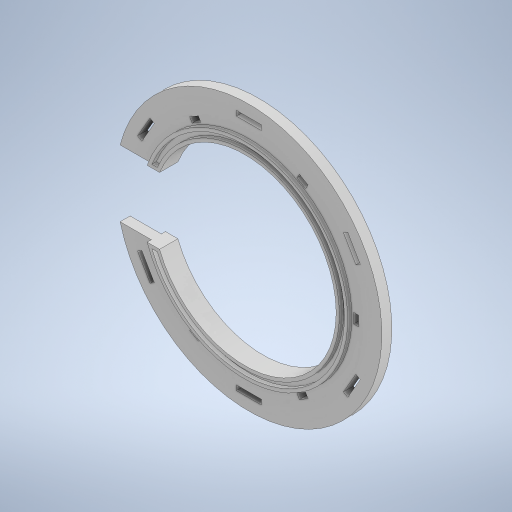
# Autodesk Inventor part: [3DP]back_cir_hold_final
Saved by Autodesk Inventor 2024 (Build 280153000, 153)
## iProperties
Created: 2024-03-23
Part Number: [3DP]back_cir_hold_final
Material: Generic
Document SubType Name: Modeling
Designer: op04o
Density: 1 g/cm^3
Appearance: Default
Author: op04o
Autodesk Inventor part; units mm, degrees
ref_plane "YZ Plane" through (0, 0, 0) normal (1, 0, 0) x (0, 1, 0)
ref_plane "XZ Plane" through (0, 0, 0) normal (0, 1, 0) x (-1, 0, 0)
ref_plane "XY Plane" through (0, 0, 0) normal (0, 0, 1) x (1, 0, 0)
sketch "Sketch1" plane through (0, 0, 0) normal (0, 0, 1) x (1, 0, 0)
  circle A0 centre (0, 0) radius 80
  circle A1 centre (0, 0) radius 55
  line L0 (-7.5, 73) -> (7.5, 73)
  line L1 (7.5, 73) -> (7.5, 70)
  line L2 (7.5, 70) -> (-7.5, 70)
  line L3 (-7.5, 70) -> (-7.5, 73)
  line L4 (-66.9699, 30.0048) -> (-59.4699, 42.9952)
  line L5 (-59.4699, 42.9952) -> (-56.8718, 41.4952)
  line L6 (-56.8718, 41.4952) -> (-64.3718, 28.5048)
  line L7 (-64.3718, 28.5048) -> (-66.9699, 30.0048)
  line L8 (-59.4699, -42.9952) -> (-66.9699, -30.0048)
  line L9 (-66.9699, -30.0048) -> (-64.3718, -28.5048)
  line L10 (-64.3718, -28.5048) -> (-56.8718, -41.4952)
  line L11 (-56.8718, -41.4952) -> (-59.4699, -42.9952)
  line L12 (7.5, -73) -> (-7.5, -73)
  line L13 (-7.5, -73) -> (-7.5, -70)
  line L14 (-7.5, -70) -> (7.5, -70)
  line L15 (7.5, -70) -> (7.5, -73)
  line L16 (66.9699, -30.0048) -> (59.4699, -42.9952)
  line L17 (59.4699, -42.9952) -> (56.8718, -41.4952)
  line L18 (56.8718, -41.4952) -> (64.3718, -28.5048)
  line L19 (64.3718, -28.5048) -> (66.9699, -30.0048)
  line L20 (59.4699, 42.9952) -> (66.9699, 30.0048)
  line L21 (66.9699, 30.0048) -> (64.3718, 28.5048)
  line L22 (64.3718, 28.5048) -> (56.8718, 41.4952)
  line L23 (56.8718, 41.4952) -> (59.4699, 42.9952)
  line L24 (-58.1708, 43.7452) -> (-43.1708, 43.7452)
  line L25 (-43.1708, 43.7452) -> (-43.1708, 40.7452)
  line L26 (-43.1708, 40.7452) -> (-58.1708, 40.7452)
  line L27 (-58.1708, 40.7452) -> (-58.1708, 43.7452)
  line L28 (-58.1708, -40.7452) -> (-43.1708, -40.7452)
  line L29 (-43.1708, -40.7452) -> (-43.1708, -43.7452)
  line L30 (-43.1708, -43.7452) -> (-58.1708, -43.7452)
  line L31 (-58.1708, -43.7452) -> (-58.1708, -40.7452)
  line L32 (0, 20) -> (-100, 20)
  line L33 (-100, 20) -> (-100, -20)
  line L34 (-100, -20) -> (0, -20)
  line L35 (0, -20) -> (0, 20)
  point P0 (0, 73)
  point P1 (7.5, 71.5)
  point P2 (0, 70)
  point P3 (-63.2199, 36.5)
  point P4 (-58.1708, 42.2452)
  point P5 (-60.6218, 35)
  point P6 (-63.2199, -36.5)
  point P7 (-65.6708, -29.2548)
  point P8 (-60.6218, -35)
  point P9 (0, -73)
  point P10 (-7.5, -71.5)
  point P11 (0, -70)
  point P12 (63.2199, -36.5)
  point P13 (58.1708, -42.2452)
  point P14 (60.6218, -35)
  point P15 (63.2199, 36.5)
  point P16 (65.6708, 29.2548)
  point P17 (60.6218, 35)
  point P18 (-58.1708, 42.2452)
  point P19 (-58.1708, -42.2452)
  point P20 (-51.2348, -20)
  point P21 (-77.4597, -20)
  point P22 (-77.4597, 20)
  point P23 (-51.2348, 20)
  dimension "d0" = 160
  dimension "d1" = 110
  dimension "d2" = 15
  dimension "d3" = 3
  dimension "d11" = 70
  dimension "d14" = 360
  dimension "d18" = 15
  dimension "d19" = 3
  dimension "d20" = 15
  dimension "d21" = 3
  dimension "d22" = 40
  dimension "d23" = 100
  constraints: 72 end point, 8 midpoint, 8 parallel, 4 horizontal, 4 perpendicular, 3 coincident, 2 centre point, 1 vertical alignment, 67 other
  measures "d0" diameter of A0
  measures "d1" diameter of A1
  measures "d2" distance of L1.end L2.end
  measures "d3" distance of L0.end L1.end
  measures "d11" distance of point (0, 0) point (0, 70)
  measures "d18" distance of L24.start L24.end
  measures "d19" distance of L24.end L25.end
  measures "d20" distance of L28.start L28.end
  measures "d21" distance of L30.end L28.start
  measures "d22" distance of L32.end L33.end
  measures "d23" distance of L32.start L32.end
extrude "Extrusion2" add sketch "Sketch1" along normal blind 6 contours A0 L34 A1 L32 | L27 L24 L25 L26 L6 L5 | L11 L10 L28 L29 L30 L31 picked at (16.7927, -65.9701)
sketch "草圖2" plane through (0, 0, 6) normal (0, 0, 1) x (1, 0, 0)
  arc A0 (-51.2348, -20) -> (-51.2348, 20) centre (0, 0) ccw projected
  circle A1 centre (0, 0) radius 55
  circle A2 centre (0, 0) radius 57
  circle A3 centre (0, 0) radius 60
  circle A4 centre (0, 0) radius 62
  arc A5 (-77.4597, -20) -> (-77.4597, 20) centre (0, 0) ccw projected
  line L0 (-51.2348, 20) -> (-77.4597, 20)
  line L1 (-51.2348, -20) -> (-77.4597, -20) projected
  line L2 (-51.2348, -20) -> (-77.4597, -20)
  line L3 (-51.2348, 20) -> (-77.4597, 20)
  line L4 (-77.4597, 20) -> (-77.4597, 22)
  line L5 (-77.4597, 22) -> (-51.2348, 22)
  line L6 (-51.2348, 22) -> (-51.2348, 20)
  line L7 (-77.4597, -20) -> (-51.2348, -20)
  line L8 (-51.2348, -20) -> (-51.2348, -22)
  line L9 (-51.2348, -22) -> (-77.4597, -22)
  line L10 (-77.4597, -22) -> (-77.4597, -20)
  point P0 (-58.6856, 20)
  point P1 (-58.6856, -20)
  point P2 (-55.8211, 22)
  point P3 (-55.8211, -22)
  point P4 (-52.5833, -22)
  point P5 (-52.5833, 22)
  dimension "d24" = 114
  dimension "d25" = 120
  dimension "d26" = 124
  dimension "d27" = 2
  dimension "d28" = 26.2249
  dimension "d29" = 2
  dimension "d30" = 26.2249
  constraints: 20 end point, 4 coincident, 4 horizontal, 4 parallel, 3 centre point, 2 perpendicular, 3 other
  measures "d24" diameter of A2
  measures "d25" diameter of A3
  measures "d26" diameter of A4
  measures "d27" distance of L3.end L4.end
  measures "d28" distance of L4.end L5.end
  measures "d29" distance of L7.end L8.end
  measures "d30" distance of L8.end L9.end
extrude "擠出3" add sketch "草圖2" against normal blind 8.5 contours L8 L9 A2 L1 | A0 L6 L5 A2 L9 L8 | L0 A2 L5 L6 | A2 L9 A3 L1 | L0 A3 L5 A2 | A3 L9 A4 L1 | L0 A4 L5 A3 | A3 L5 A4 L9
extrude "擠出4" add sketch "草圖2" along normal blind 2.5 contours L8 L9 A2 L1 | A0 L6 L5 A2 L9 L8 | L0 A2 L5 L6 | A2 L9 A3 L1 | L0 A3 L5 A2 | A3 L9 A4 L1 | L0 A4 L5 A3 | A3 L5 A4 L9
sketch "草圖3" plane through (0, 0, 6) normal (0, 0, 1) x (1, 0, 0)
  line L0 (63, 3) -> (66, 3)
  line L1 (66, 3) -> (66, -3)
  line L2 (66, -3) -> (63, -3)
  line L3 (63, -3) -> (63, 3)
  line L4 (28.9019, 56.0596) -> (30.4019, 58.6577)
  line L5 (30.4019, 58.6577) -> (35.5981, 55.6577)
  line L6 (35.5981, 55.6577) -> (34.0981, 53.0596)
  line L7 (34.0981, 53.0596) -> (28.9019, 56.0596)
  line L8 (-34.0981, 53.0596) -> (-35.5981, 55.6577)
  line L9 (-35.5981, 55.6577) -> (-30.4019, 58.6577)
  line L10 (-30.4019, 58.6577) -> (-28.9019, 56.0596)
  line L11 (-28.9019, 56.0596) -> (-34.0981, 53.0596)
  line L12 (-63, -3) -> (-66, -3)
  line L13 (-66, -3) -> (-66, 3)
  line L14 (-66, 3) -> (-63, 3)
  line L15 (-63, 3) -> (-63, -3)
  line L16 (-28.9019, -56.0596) -> (-30.4019, -58.6577)
  line L17 (-30.4019, -58.6577) -> (-35.5981, -55.6577)
  line L18 (-35.5981, -55.6577) -> (-34.0981, -53.0596)
  line L19 (-34.0981, -53.0596) -> (-28.9019, -56.0596)
  line L20 (34.0981, -53.0596) -> (35.5981, -55.6577)
  line L21 (35.5981, -55.6577) -> (30.4019, -58.6577)
  line L22 (30.4019, -58.6577) -> (28.9019, -56.0596)
  line L23 (28.9019, -56.0596) -> (34.0981, -53.0596)
  point P0 (0, 0)
  point P1 (63, 0)
  point P2 (31.5, 54.5596)
  point P3 (-31.5, 54.5596)
  point P4 (-63, 0)
  point P5 (-31.5, -54.5596)
  point P6 (31.5, -54.5596)
  dimension "d42" = 3
  dimension "d43" = 6
  dimension "d44" = 63
  dimension "d47" = 360
  constraints: 48 end point, 2 parallel, 1 horizontal, 1 horizontal alignment, 1 midpoint, 1 perpendicular, 55 other
  measures "d42" distance of L1.end L2.end
  measures "d43" distance of L0.end L1.end
  measures "d44" distance from line of point (0, 0) L3
extrude "擠出5" cut sketch "草圖3" against normal through all contours L0 L1 L2 L3 | L4 L5 L6 L7 | L8 L9 L10 L11 | L16 L17 L18 L19 | L20 L21 L22 L23
body "Solid2"
